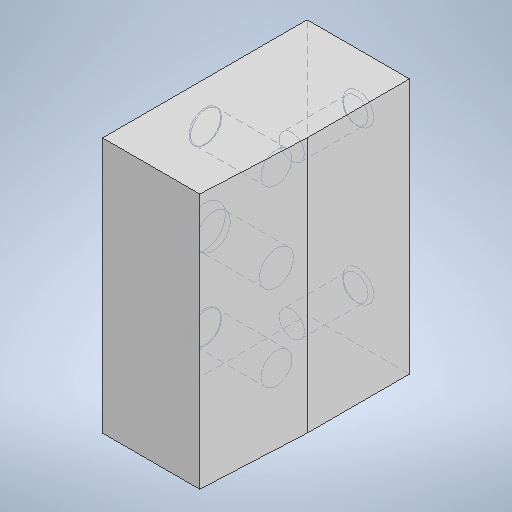
# Autodesk Inventor part: ER_Positionierungseinheit_Backe_int
Saved by Autodesk Inventor 2025.1 (Build 291241000, 241)
## iProperties
Created: 2025-05-23
Part Number: ER_Positionierungseinheit_Backe_int
Material: Generic
Document SubType Name: Modeling
Designer: Erik
Density: 1 g/cm^3
Appearance: Default
Author: Erik
Autodesk Inventor part; units mm, degrees
ref_plane "YZ Plane" through (0, 0, 0) normal (1, 0, 0) x (0, 1, 0)
ref_plane "XZ Plane" through (0, 0, 0) normal (0, 1, 0) x (-1, 0, 0)
ref_plane "XY Plane" through (0, 0, 0) normal (0, 0, 1) x (1, 0, 0)
sketch "Sketch2" plane through (0, 0, 0) normal (0, 1, 0) x (-1, 0, 0)
  line L0 (-10, 25) -> (10, 25)
  line L1 (10, 25) -> (10, -25)
  line L2 (10, -25) -> (-10, -25)
  line L3 (-10, -25) -> (-10, 25)
  line L4 (-10, 25) -> (10, -25) construction
  line L5 (10, 25) -> (-10, -25) construction
  point P0 (0, 0)
  dimension "d0" = 50
  dimension "d1" = 20
  constraints: 12 end point, 2 midpoint, 2 parallel, 1 horizontal, 1 perpendicular
  measures "d0" distance of L0.end L1.end
  measures "d1" distance of L1.end L2.end
extrude "Extrusion1" add sketch "Sketch2" along normal blind 40
sketch "Sketch3" plane through (-10, 0, 25) normal (0, 0, 1) x (1, 0, 0)
  line L0 (20, 0) -> (20, 40) projected
  line L1 (20, 40) -> (20, 20)
  line L2 (0, 40) -> (20, 40) projected
  line L3 (20, 20) -> (19, 0)
  line L4 (20, 0) -> (0, 0) projected
  line L5 (19, 0) -> (20, 0)
  line L6 (20, 0) -> (20, 20)
  point P0 (10, 0)
  dimension "d4" = 20
  dimension "d5" = 1
  constraints: 8 end point, 1 collinear, 1 midpoint, 1 perpendicular, 1 point on line
  measures "d4" distance from line of L2 L1.end
  measures "d5" distance from line of L0 L3.end
extrude "Extrusion2" cut sketch "Sketch3" against normal through all
sketch "Sketch4" plane through (-10, 0, -25) normal (-1, 0, 0) x (0, 0, 1)
  line L0 (0, 0) -> (0, 40) projected
  line L1 (50, 0) -> (50, 40) projected
  line L2 (25, 0) -> (25, 40) construction
  line L3 (50, 40) -> (0, 40) projected
  line L4 (0, 20) -> (50, 20) construction
  line L5 (0, 0) -> (50, 0) projected
  point P0 (8, 20)
  point P1 (42, 20)
  point P2 (25, 20)
  dimension "d8" = 8
  dimension "d9" = 8
  dimension "d10" = 20
  constraints: 5 midpoint, 4 end point, 2 point on line, 1 perpendicular
  measures "d8" distance from line of L0 point (8, 20)
  measures "d9" distance from line of L1 point (42, 20)
  measures "d10" distance between parallel lines of L5 L4
hole "Hole1" at (-10, 20, -17) at (-10, 20, 17) direction (1, 0, 0) diameter 6 depth 14 tip angle 118 countersink diameter 6.2 countersink angle 45
hole "Hole2" at (-10, 20, 0) direction (1, 0, 0) diameter 6.647 depth 14 tip angle 118 countersink diameter 8 countersink angle 45 thread size "M8x1.25" class "6H" standard "ISO Metric profile"
sketch "Sketch5" plane through (0, 40, 0) normal (0, 1, 0) x (1, 0, 0)
  line L0 (10, 25) -> (-10, 25) projected
  line L1 (-10, 25) -> (-10, -25) projected
  line L2 (-10, -25) -> (10, -25) projected
  line L3 (10, -25) -> (10, 25) projected
  line L4 (0, 25) -> (0, -25) construction
  point P0 (0, 0)
  point P1 (0, 15)
  point P2 (0, -15)
  point P3 (0, 0)
  dimension "d25" = 15
  dimension "d26" = 15
  constraints: 3 midpoint, 2 end point, 2 point on line
  measures "d25" distance of point (0, 0) point (0, -15)
  measures "d26" distance of point (0, 15) point (0, 0)
hole "Hole3" at (0, 40, -15) at (0, 40, 15) direction (0, -1, 0) diameter 4.917 depth 13 tip angle 118 countersink diameter 6 countersink angle 90 thread size "M6x1" class "6H" standard "ISO Metric profile"
equation "\"d0\" = Länge_Backe"
equation "\"d1\" = Breite_Backe"
equation "\"d2\" = Höhe_Backe"
equation "\"d4\" = Absatz_Höhe"
equation "\"d5\" = 0.5 * Max_Versatz"
equation "\"d8\" = d9"
equation "\"d9\" = Abstand_Bolzen"
equation "\"d10\" = Höhe_Schrauben"
equation "\"d11\" = Bolzen_Durchmesser"
equation "\"d25\" = 0.5 * Abstand_Bohrung_Vertikale_halterung"
equation "\"d26\" = d25"
equation "\"Breite_Backe\" = 20"
equation "\"Höhe_Backe\" = 40"
equation "\"Länge_Backe\" = 50"
equation "\"Absatz_Höhe\" = 20"
equation "\"Max_Versatz\" = 2"
equation "\"Abstand_Bolzen\" = 8"
equation "\"Höhe_Schrauben\" = 20"
equation "\"Bolzen_Durchmesser\" = 6"
equation "\"Abstand_Bohrung_Vertikale_halterung\" = 30"
body "Solid1"
